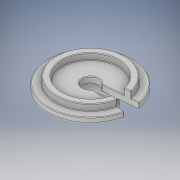
# Autodesk Inventor part: Spring Cup
Saved by Autodesk Inventor 2019 (Build 230136000, 136)
## iProperties
Created: 2019-11-29
Part Number: Spring Cup
Material: Generic
Document SubType Name: Modeling
Designer: Jopa
Density: 1 g/cm^3
Appearance: Default
Author: Jopa
Autodesk Inventor part; units mm, degrees
ref_plane "YZ Plane" through (0, 0, 0) normal (1, 0, 0) x (0, 1, 0)
ref_plane "XZ Plane" through (0, 0, 0) normal (0, 1, 0) x (-1, 0, 0)
ref_plane "XY Plane" through (0, 0, 0) normal (0, 0, 1) x (1, 0, 0)
sketch "Sketch1" plane through (0, 0, 0) normal (0, 0, 1) x (1, 0, 0)
  line L0 (0, -3.556) -> (0, 3.556) projected
  line L1 (-10.287, 0) -> (1.7145, 0) projected
  line L2 (-1.651, 0) -> (-1.651, 1.27)
  line L3 (-1.651, 1.27) -> (-5.715, 1.27)
  line L4 (-5.715, 1.27) -> (-5.715, 2.54)
  line L5 (-5.715, 2.54) -> (-6.985, 2.54)
  line L6 (-6.985, 2.54) -> (-6.985, 1.27)
  line L7 (-6.985, 1.27) -> (-8.5725, 1.27)
  line L8 (-8.5725, 1.27) -> (-8.5725, 0)
  line L9 (-8.5725, 0) -> (-4.2545, 0)
  line L10 (-4.2545, -2.54) -> (-4.2545, 0)
  line L11 (-4.2545, -2.54) -> (-2.9845, -2.54)
  line L12 (-2.9845, -2.54) -> (-2.9845, 0)
  line L13 (-1.651, 0) -> (-2.9845, 0)
  point P0 (0, 0)
  dimension "d0" = 3.302
  dimension "d1" = 1.27
  dimension "d2" = 11.43
  dimension "d3" = 1.27
  dimension "d4" = 2.54
  dimension "d5" = 1.27
  dimension "d6" = 17.145
  dimension "d7" = 5.969
  constraints: 24 end point, 8 perpendicular, 4 point on line, 2 collinear, 2 horizontal, 1 vertical
  measures "d0" diameter of L2 L0
  measures "d1" distance of L2.start L2.end
  measures "d2" diameter of L4 L0
  measures "d3" distance between parallel lines of L4 L6
  measures "d4" distance of L10.start L9.end
  measures "d5" distance of L10.start L11.end
  measures "d6" diameter of L8 L0
  measures "d7" diameter of L12 L0
revolve "Revolution1" add sketch "Sketch1" angle 360 about axis through (0, -10, 0) along (0, 1, 0)
fillet "Fillet1" radius 0.381 3 edges at (4.2545, -2.54, 0) (4.2545, 0, 0) (8.5725, 0, 0)
sketch "Sketch2" plane through (0, 1.27, 0) normal (0, 1, 0) x (1, 0, 0)
  circle A0 centre (0, 0) radius 8.5725 construction
  circle A1 centre (0, 0) radius 6.985 construction
  circle A2 centre (0, 0) radius 5.715 construction
  circle A3 centre (0, 0) radius 1.651 construction
  line L0 (0, -0.7937) -> (0, 0.7937)
  line L1 (0, -0.7937) -> (8.5725, -1.5437)
  line L2 (8.5725, -1.5437) -> (8.5725, 1.5437)
  line L3 (8.5725, 1.5437) -> (0, 0.7937)
  circle A4 centre (0, 0) radius 8.5725 projected
  point P0 (8.5725, 0)
  dimension "d10" = 1.5875
  dimension "d11" = 10
  constraints: 8 end point, 2 midpoint, 2 vertical, 1 coincident, 1 horizontal alignment, 1 tangent
  measures "d10" distance of L0.start L0.end
  measures "d11" angle of L3 L1
extrude "Extrusion1" cut sketch "Sketch2" along normal through all both and the other way through all contours L0 L3 A4 L1 | A4 L2 L1 | L3 L2 A4 picked at (2.8575, 0)
fillet "Fillet2" radius 0.127 8 edges at (-8.5725, 1.27, 0) (-6.985, 1.27, 0) (-6.985, 2.54, 0) (-5.715, 2.54, 0) (-5.715, 1.27, 0) (-1.651, 1.27, 0) (-1.651, 0, 0) (-2.9845, 0, 0)
fillet "Fillet3" radius 0.127 46 edges at (6.8821, 1.3071, 1.3959) (6.8448, 1.905, 1.3926) (6.8075, 2.5028, 1.3893) (6.2074, 2.54, 1.3368) (5.607, 2.5028, 1.2843) (5.5696, 1.905, 1.281) (5.5322, 1.3072, 1.2778) (3.4797, 1.27, 1.0982) (1.417, 1.2329, 0.9177) (1.3749, 0.635, 0.914) (1.417, 0.0371, 0.9177) (2.092, 0, 0.9768) (2.7595, -0.0372, 1.0352) (2.798, -1.3335, 1.0385) (8.3973, 1.2328, 1.5284) (8.4346, 0.762, 1.5317) (8.3229, 0.1116, 1.5219) (6.2673, 0, 1.3421) (4.2088, -0.1115, 1.162) (4.0955, -1.27, 1.1521) (3.9822, -2.4286, 1.1421) (3.2533, -2.54, 1.0784) (7.6398, 1.27, 1.4621) (8.3973, 1.2328, -1.5284) (8.4346, 0.762, -1.5317) (8.3229, 0.1116, -1.5219) (6.2673, 0, -1.3421) (4.2088, -0.1115, -1.162) (4.0955, -1.27, -1.1521) (3.9822, -2.4286, -1.1421) (3.2533, -2.54, -1.0784) (6.8821, 1.3072, -1.3959) (6.8448, 1.905, -1.3926) (6.8074, 2.5029, -1.3893) (6.2074, 2.54, -1.3368) (5.607, 2.5028, -1.2843) (5.5696, 1.905, -1.281) (5.5321, 1.3071, -1.2777) (3.4797, 1.27, -1.0982) (1.417, 1.2329, -0.9177) (1.3749, 0.635, -0.914) (1.417, 0.0371, -0.9177) (2.092, 0, -0.9768) (2.7595, -0.0372, -1.0352) (2.798, -1.3335, -1.0385) (7.6398, 1.27, -1.4621)
body "Solid1"
